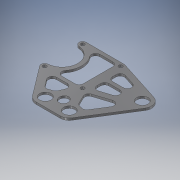
# Autodesk Inventor part: Part1
Saved by Autodesk Inventor 2018 (Build 220112000, 112)
## iProperties
Created: 2018-10-10
Part Number: Part1
Material: アルミニウム 2014-T4
Document SubType Name: Modeling
Designer: taka
Density: 2.8 g/cm^3
Appearance: サテン
Author: taka
Autodesk Inventor part; units mm, degrees
ref_plane "YZ Plane" through (0, 0, 0) normal (1, 0, 0) x (0, 1, 0)
ref_plane "XZ Plane" through (0, 0, 0) normal (0, 1, 0) x (-1, 0, 0)
ref_plane "XY Plane" through (0, 0, 0) normal (0, 0, 1) x (1, 0, 0)
sketch "スケッチ1" plane through (0, 0, 0) normal (0, 0, 1) x (1, 0, 0)
  circle A0 centre (68, 27) radius 4.05
  circle A1 centre (31, -5) radius 4.05
  circle A2 centre (48, -5) radius 4.05
  circle A3 centre (68, 27) radius 6.5 construction
  circle A4 centre (31, -5) radius 6.5 construction
  circle A5 centre (48, -5) radius 6.5 construction
  line L0 (31, -11.5) -> (48, -11.5)
  line L1 (73.512, 23.555) -> (53.512, -8.445)
  arc A6 (48, -11.5) -> (53.512, -8.445) centre (48, -5) ccw
  circle A7 centre (39, 13.5) radius 1.35
  line L2 (39, 13.5) -> (39, 40.5) construction
  line L3 (39, 40.5) -> (12, 40.5) construction
  line L4 (12, 40.5) -> (12, 13.5) construction
  line L5 (12, 13.5) -> (39, 13.5) construction
  circle A8 centre (12, 13.5) radius 1.35
  circle A9 centre (12, 40.5) radius 1.35
  circle A10 centre (39, 40.5) radius 1.35
  circle A11 centre (11, 27) radius 8.5 construction
  circle A12 centre (11, 27) radius 10.5 construction
  arc A13 (0, 15.381) -> (0, 38.619) centre (11, 27) ccw construction
  line L6 (0, 15.381) -> (0, 38.619) construction
  line L7 (11, 11) -> (11, 43) construction
  line L8 (11, 43) -> (51.5, 43) construction
  line L9 (51.5, 43) -> (51.5, 11) construction
  line L10 (51.5, 11) -> (11, 11) construction
  circle A14 centre (39, 13.5) radius 2.5 construction
  circle A15 centre (39, 40.5) radius 2.5 construction
  circle A16 centre (12, 40.5) radius 2.5 construction
  circle A17 centre (12, 13.5) radius 2.5 construction
  line L11 (10.0057, 11.9924) -> (25.8149, -8.9198)
  line L12 (69.9848, 33.1896) -> (39.7634, 42.8806)
  arc A18 (25.8149, -8.9198) -> (31, -11.5) centre (31, -5) ccw
  arc A19 (12, 16) -> (10.0057, 11.9924) centre (12, 13.5) ccw
  arc A20 (12, 16) -> (12, 38) centre (11, 27) ccw
  line L13 (12, 43) -> (39, 43)
  arc A21 (39.7634, 42.8806) -> (39, 43) centre (39, 40.5) ccw
  arc A22 (73.512, 23.555) -> (69.9848, 33.1896) centre (68, 27) ccw
  arc A23 (12, 43) -> (12, 38) centre (12, 40.5) ccw
  point P0 (0, 0)
  point P1 (62.8293, 30.9388)
  point P2 (24.5, -5)
  point P3 (1.5716, 22.3787)
  point P4 (39, 11)
  dimension "d60" = 21
  dimension "d17" = 8.1
  dimension "d21" = 5
  dimension "d24" = 17
  dimension "d26" = 20
  dimension "d27" = 13
  dimension "d55" = 2.7
  dimension "d56" = 27
  dimension "d57" = 27
  dimension "d58" = 17
  dimension "d59" = 1
  dimension "d61" = 32
  dimension "d62" = 13.5
  dimension "d63" = 12
  dimension "d64" = 51.5
  dimension "d65" = 5
  dimension "d66" = 57
  dimension "d67" = 32
  dimension "d68" = 32
  dimension "d69" = 20
  constraints: 31 point on circle, 28 end point, 22 centre point, 19 coincident, 9 equal radius, 9 tangent, 6 point on line, 4 parallel, 2 horizontal, 2 perpendicular, 1 vertical alignment, 7 other
  measures "d17" diameter of A0
  measures "d21" vertical distance of A1.centre point (0, 0)
  measures "d24" distance of A2.centre A1.centre
  measures "d26" horizontal distance of A2.centre A0.centre
  measures "d27" diameter of A3
  measures "d55" diameter of A7
  measures "d56" distance of L5.start L3.end
  measures "d57" distance of L3.end L2.end
  measures "d58" diameter of A11
  measures "d59" distance from line of L4 A11.centre
  measures "d61" diameter of A13
  measures "d62" distance from line of A11.centre L5
  measures "d63" distance between parallel lines of L4 L6
  measures "d64" distance between parallel lines of L9 L6
  measures "d65" diameter of A15
  measures "d66" distance of A0.centre A13.centre
  measures "d67" vertical distance of A0.centre A2.centre
  measures "d68" vertical distance of point (11, 27) A1.centre
  measures "d69" horizontal distance of A1.centre A13.centre
extrude "押し出し1" add sketch "スケッチ1" along normal blind 2
sketch "スケッチ5" plane through (0, 0, 2) normal (0, 0, 1) x (1, 0, 0)
  circle A0 centre (12, 40.5) radius 1.35 projected
  circle A1 centre (39, 40.5) radius 1.35 projected
  circle A2 centre (39, 13.5) radius 1.35 projected
  circle A3 centre (12, 13.5) radius 1.35 projected
  circle A4 centre (31, -5) radius 4.05 projected
  circle A5 centre (48, -5) radius 4.05 projected
  circle A6 centre (68, 27) radius 4.05 projected
  line L0 (39, 43) -> (12, 43) projected
  circle A7 centre (12, 40.5) radius 2.5 construction
  circle A8 centre (39, 40.5) radius 2.5 construction
  circle A9 centre (39, 13.5) radius 2.5 construction
  circle A10 centre (12, 13.5) radius 2.5 construction
  circle A11 centre (31, -5) radius 6.5 construction
  circle A12 centre (48, -5) radius 6.5 construction
  circle A13 centre (68, 27) radius 6.5 construction
  arc A14 (73.512, 23.555) -> (69.9848, 33.1896) centre (68, 27) ccw projected
  line L1 (14.5, 40.5) -> (36.5, 40.5)
  line L2 (36.5, 40.5) -> (36.5, 13.5)
  line L3 (14.5, 13.5) -> (36.5, 13.5)
  arc A15 (12, 16) -> (12, 38) centre (11, 27) ccw projected
  arc A16 (14.5, 13.5) -> (14.5, 40.5) centre (11, 27) ccw
  line L4 (40.4464, 38.4609) -> (42.5, 37.8024)
  line L5 (69.9848, 33.1896) -> (39.7634, 42.8806) projected
  line L6 (68, 27) -> (11, 27) construction
  line L7 (63.0499, 22.7873) -> (42.5, 16.1976)
  line L8 (42.5, 37.8024) -> (42.5, 28.25)
  line L9 (39.7634, 11.1194) -> (42.5098, 12.0001)
  arc A17 (63.0499, 31.2127) -> (61.6213, 28.25) centre (68, 27) ccw
  line L10 (39, 13.5) -> (48, -5) construction
  line L11 (39, 13.5) -> (31, -5) construction
  line L12 (41.2481, 14.5937) -> (42.5098, 12.0001)
  line L13 (36.7519, 12.4063) -> (39.1337, 7.5105)
  line L14 (41.2946, 12.5077) -> (39.1337, 7.5105)
  line L15 (65.92, 20.8418) -> (64.8766, 19.1724)
  line L16 (53.512, -8.445) -> (73.512, 23.555) projected
  arc A18 (52.624, -0.4318) -> (47.6233, 1.4891) centre (48, -5) ccw
  line L17 (10.0057, 11.9924) -> (25.8149, -8.9198) projected
  line L18 (37.5, -5) -> (41.5, -5)
  arc A19 (43.1271, -0.6983) -> (41.5, -5) centre (48, -5) ccw
  arc A20 (37.5, -5) -> (35.6761, -0.4851) centre (31, -5) ccw
  arc A21 (31.0868, 1.4994) -> (25.9894, -0.8594) centre (31, -5) ccw
  line L19 (31, -5) -> (48, -5) construction
  line L20 (39.1337, 7.5105) -> (43.1271, -0.6983)
  line L21 (39.1337, 7.5105) -> (35.6761, -0.4851)
  line L22 (42.5098, 12.0001) -> (64.8766, 19.1724)
  line L23 (42.5098, 12.0001) -> (47.6233, 1.4891)
  line L24 (42.5, 16.1976) -> (40.4464, 15.5391)
  line L25 (42.5, 37.8024) -> (63.0499, 31.2127)
  line L26 (64.8766, 19.1724) -> (69.9848, 20.8104)
  line L27 (64.8766, 19.1724) -> (52.624, -0.4318)
  line L28 (36.0599, 11) -> (35.1952, 11)
  line L29 (36.7054, 14.4923) -> (35.1952, 11)
  line L30 (25.9894, -0.8594) -> (17.0239, 11)
  line L31 (17.0239, 11) -> (13.9943, 15.0076)
  line L32 (17.0239, 11) -> (14.4985, 11)
  line L33 (35.1952, 11) -> (17.0239, 11)
  line L34 (35.1952, 11) -> (31.0868, 1.4994)
  line L35 (61.6213, 28.25) -> (42.5, 28.25)
  line L36 (61.6213, 25.75) -> (42.5, 25.75)
  arc A22 (61.6213, 28.25) -> (61.6213, 25.75) centre (68, 27) ccw construction
  arc A23 (61.6213, 25.75) -> (63.0499, 22.7873) centre (68, 27) ccw
  line L37 (42.5, 28.25) -> (42.5, 25.75) construction
  line L38 (42.5, 25.75) -> (42.5, 16.1976)
  point P0 (0, 0)
  dimension "d71" = 4
  dimension "d73" = 5
  dimension "d75" = 5
  dimension "d81" = 6
  dimension "d82" = 2.5
  dimension "d83" = 5
  dimension "d84" = 5
  dimension "d85" = 2.5
  constraints: 70 end point, 34 point on circle, 22 parallel, 14 centre point, 12 coincident, 4 equal radius, 4 horizontal, 3 vertical, 2 perpendicular, 2 point on line, 2 tangent, 1 collinear, 1 concentric, 17 other
  measures "d71" distance between parallel lines of L5 L4
  measures "d73" distance between parallel lines of L12 L13
  measures "d75" distance between parallel lines of L16 L15
  measures "d81" distance between parallel lines of L2 L8
  measures "d82" distance between parallel lines of L3 L28
  measures "d83" distance between parallel lines of L29 L21
  measures "d84" distance between parallel lines of L17 L30
  measures "d85" distance between parallel lines of L36 L35
extrude "押し出し3" cut sketch "スケッチ5" against normal through all contours L1 L2 L29 L3 L31 A16 | L31 L3 A16 | L2 L3 L29 | L33 L34 A21 L30 | L7 L38 L36 A23 | L25 A17 L35 L8 | A18 L23 L22 L27 | A20 L21 L20 A19 L18
fillet "フィレット2" radius 3 25 edges at (36.5, 13.5, 1) (39.1337, 7.5105, 1) (42.5098, 12.0001, 1) (35.6761, -0.4851, 1) (37.5, -5, 1) (43.1271, -0.6983, 1) (41.5, -5, 1) (47.6233, 1.4891, 1) (52.624, -0.4318, 1) (64.8766, 19.1724, 1) (63.0499, 22.7873, 1) (63.0499, 31.2127, 1) (42.5, 37.8024, 1) (36.5, 40.5, 1) (31.0868, 1.4994, 1) (25.9894, -0.8594, 1) (42.5, 16.1976, 1) (14.5, 13.5, 1) (14.5, 40.5, 1) (35.1952, 11, 1) (17.0239, 11, 1) (42.5, 25.75, 1) (42.5, 28.25, 1) (61.6213, 28.25, 1) (61.6213, 25.75, 1)
equation "\"d62\" = 0.5 * d56"
equation "\"d45\" = d44"
equation "\"d44\" = 6"
